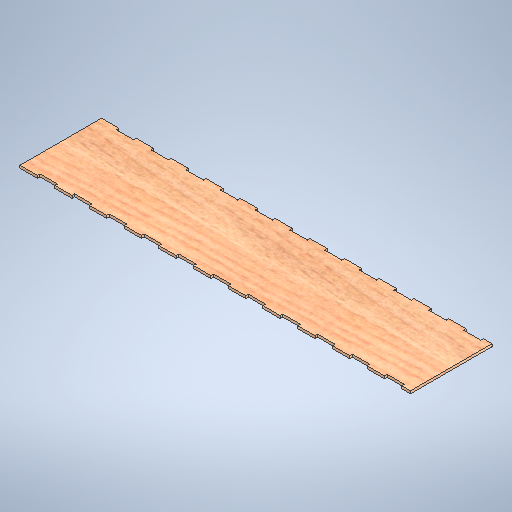
# Autodesk Inventor part: Part2 box
Saved by Autodesk Inventor 2025.3 (Build 293356000, 356)
## iProperties
Created: 2026-04-05
Part Number: Part2 box
Material: Wood (Birch)
Document SubType Name: Modeling
Designer: logien
Density: 0.55 g/cm^3
Appearance: Birch - Natural Polished
Author: logien
Autodesk Inventor part; units mm, degrees
ref_plane "YZ Plane" through (0, 0, 0) normal (1, 0, 0) x (0, 1, 0)
ref_plane "XZ Plane" through (0, 0, 0) normal (0, 1, 0) x (-1, 0, 0)
ref_plane "XY Plane" through (0, 0, 0) normal (0, 0, 1) x (1, 0, 0)
sketch "Sketch1" plane through (0, 0, 0) normal (0, 1, 0) x (-1, 0, 0)
  line L0 (0, 0) -> (0, -88)
  line L1 (30, -88) -> (30, -91)
  line L2 (30, -91) -> (50, -91)
  line L3 (50, -91) -> (50, -88)
  line L4 (50, -88) -> (70, -88)
  line L5 (70, -88) -> (70, -91)
  line L6 (70, -91) -> (90, -91)
  line L7 (90, -91) -> (90, -88)
  line L8 (90, -88) -> (110, -88)
  line L9 (110, -88) -> (110, -91)
  line L10 (110, -91) -> (130, -91)
  line L11 (130, -91) -> (130, -88)
  line L12 (130, -88) -> (150, -88)
  line L13 (150, -88) -> (150, -91)
  line L14 (150, -91) -> (170, -91)
  line L15 (170, -91) -> (170, -88)
  line L16 (170, -88) -> (190, -88)
  line L17 (190, -88) -> (190, -91)
  line L18 (190, -91) -> (210, -91)
  line L19 (210, -91) -> (210, -88)
  line L20 (210, -88) -> (230, -88)
  line L21 (230, -88) -> (230, -91)
  line L22 (230, -91) -> (250, -91)
  line L23 (250, -91) -> (250, -88)
  line L24 (250, -88) -> (270, -88)
  line L25 (270, -88) -> (270, -91)
  line L26 (270, -91) -> (290, -91)
  line L27 (290, -91) -> (290, -88)
  line L28 (290, -88) -> (310, -88)
  line L29 (310, -88) -> (310, -91)
  line L30 (310, -91) -> (330, -91)
  line L31 (330, -91) -> (330, -88)
  line L32 (330, -88) -> (350, -88)
  line L33 (350, -88) -> (350, -91)
  line L34 (350, -91) -> (370, -91)
  line L35 (370, -91) -> (370, -88)
  line L36 (370, -88) -> (390, -88)
  line L37 (390, -88) -> (390, -91)
  line L38 (390, -91) -> (410, -91)
  line L39 (410, -91) -> (410, -88)
  line L40 (410, -88) -> (430, -88)
  line L41 (430, -88) -> (430, -91)
  line L42 (0, -44) -> (10, -44)
  line L43 (30, 0) -> (30, 3)
  line L44 (30, 3) -> (50, 3)
  line L45 (50, 3) -> (50, 0)
  line L46 (50, 0) -> (70, 0)
  line L47 (70, 0) -> (70, 3)
  line L48 (70, 3) -> (90, 3)
  line L49 (90, 3) -> (90, 0)
  line L50 (90, 0) -> (110, 0)
  line L51 (110, 0) -> (110, 3)
  line L52 (110, 3) -> (130, 3)
  line L53 (130, 3) -> (130, 0)
  line L54 (130, 0) -> (150, 0)
  line L55 (150, 0) -> (150, 3)
  line L56 (150, 3) -> (170, 3)
  line L57 (170, 3) -> (170, 0)
  line L58 (170, 0) -> (190, 0)
  line L59 (190, 0) -> (190, 3)
  line L60 (190, 3) -> (210, 3)
  line L61 (210, 3) -> (210, 0)
  line L62 (210, 0) -> (230, 0)
  line L63 (230, 0) -> (230, 3)
  line L64 (230, 3) -> (250, 3)
  line L65 (250, 3) -> (250, 0)
  line L66 (250, 0) -> (270, 0)
  line L67 (270, 0) -> (270, 3)
  line L68 (270, 3) -> (290, 3)
  line L69 (290, 3) -> (290, 0)
  line L70 (290, 0) -> (310, 0)
  line L71 (310, 0) -> (310, 3)
  line L72 (310, 3) -> (330, 3)
  line L73 (330, 3) -> (330, 0)
  line L74 (330, 0) -> (350, 0)
  line L75 (350, 0) -> (350, 3)
  line L76 (350, 3) -> (370, 3)
  line L77 (370, 3) -> (370, 0)
  line L78 (370, 0) -> (390, 0)
  line L79 (390, 0) -> (390, 3)
  line L80 (390, 3) -> (410, 3)
  line L81 (410, 3) -> (410, 0)
  line L82 (410, 0) -> (430, 0)
  line L83 (430, -91) -> (450, -91)
  line L84 (430, 0) -> (430, 3)
  line L85 (430, 3) -> (450, 3)
  line L86 (450, 3) -> (450, -91)
  line L87 (30, -88) -> (10, -88)
  line L88 (10, -88) -> (10, -91)
  line L89 (10, -91) -> (0, -91)
  line L90 (0, -91) -> (0, -88)
  line L91 (30, 0) -> (10, 0)
  line L92 (10, 0) -> (10, 3)
  line L93 (10, 3) -> (0, 3)
  line L94 (0, 3) -> (0, 0)
  dimension "d0" = 88
  dimension "d26" = 3
  dimension "d27" = 20
  dimension "d28" = 20
  dimension "d29" = 20
  dimension "d30" = 20
  dimension "d31" = 20
  dimension "d32" = 20
  dimension "d33" = 20
  dimension "d34" = 20
  dimension "d35" = 20
  dimension "d36" = 20
  dimension "d37" = 20
  dimension "d38" = 20
  dimension "d39" = 20
  dimension "d40" = 20
  dimension "d41" = 20
  dimension "d42" = 20
  dimension "d43" = 20
  dimension "d44" = 20
  dimension "d45" = 20
  dimension "d46" = 20
  dimension "d48" = 10
  dimension "d59" = 20
  dimension "d64" = 3
  dimension "d65" = 3
  dimension "d66" = 3
  dimension "d67" = 3
  dimension "d68" = 20
  dimension "d69" = 20
  dimension "d70" = 3
  constraints: 190 end point, 61 point on line, 41 symmetric about line, 31 perpendicular, 6 horizontal, 3 vertical, 1 collinear, 1 midpoint
  measures "d0" distance of L0.start L0.end
  measures "d26" distance of L1.start L1.end
  measures "d27" distance of L1.end L2.end
  measures "d28" distance of L3.end L4.end
  measures "d29" distance of L5.end L6.end
  measures "d30" distance of L7.end L8.end
  measures "d31" distance of L9.end L10.end
  measures "d32" distance of L11.end L12.end
  measures "d33" distance of L13.end L14.end
  measures "d34" distance of L15.end L16.end
  measures "d35" distance of L17.end L18.end
  measures "d36" distance of L19.end L20.end
  measures "d37" distance of L21.end L22.end
  measures "d38" distance of L23.end L24.end
  measures "d39" distance of L25.end L26.end
  measures "d40" distance of L27.end L28.end
  measures "d41" distance of L29.end L30.end
  measures "d42" distance of L31.end L32.end
  measures "d43" distance of L33.end L34.end
  measures "d44" distance of L35.end L36.end
  measures "d45" distance of L37.end L38.end
  measures "d46" distance of L39.end L40.end
  measures "d48" distance of L42.start L42.end
  measures "d59" distance of L41.end L83.end
  measures "d64" distance of L40.end L41.end
  measures "d65" distance of L24.end L25.end
  measures "d66" distance of L8.end L9.end
  measures "d67" distance of L82.end L84.end
  measures "d68" distance of L1.start L87.end
  measures "d69" distance of L43.start L91.end
  measures "d70" distance of L91.end L92.end
extrude "Extrusion1" add sketch "Sketch1" along normal blind 3
body "Solid1"
